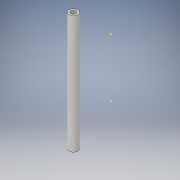
# Autodesk Inventor part: stem1
Saved by Autodesk Inventor 2019 (Build 230136000, 136)
## iProperties
Created: 2020-02-19
Part Number: stem1
Material: Generic
Document SubType Name: Modeling
Designer: FCI-L628
Density: 1 g/cm^3
Appearance: Default
Author: FCI-L628
Autodesk Inventor part; units mm, degrees
ref_plane "YZ Plane" through (0, 0, 0) normal (1, 0, 0) x (0, 1, 0)
ref_plane "XZ Plane" through (0, 0, 0) normal (0, 1, 0) x (-1, 0, 0)
ref_plane "XY Plane" through (0, 0, 0) normal (0, 0, 1) x (1, 0, 0)
sketch "Sketch1" plane through (0, 0, 0) normal (0, 0, 1) x (1, 0, 0)
  point P0 (0, 0)
sketch "Sketch2" plane through (0, 0, 0) normal (0, 0, 1) x (1, 0, 0)
  line L0 (-9.2557, 14.4492) -> (-8.1759, 14.4492)
  line L1 (-8.1759, 14.4492) -> (-8.1759, -14.7063)
  line L2 (-8.1759, -14.7063) -> (-9.2557, -14.7063)
  line L3 (-9.2557, -14.7063) -> (-9.2557, 14.4492)
  point P0 (0, 0)
  constraints: 8 end point, 2 parallel, 1 horizontal, 1 perpendicular
revolve "Revolution1" add sketch "Sketch2" angle 360 about axis through (-9.2557, -14.7063, 0) along (0, 1, 0)
sketch "Sketch3" plane through (-9.2557, 14.4492, 0) normal (0, 1, 0) x (1, 0, 0)
  circle A0 centre (0, 0) radius 1.0798 projected
  circle A1 centre (0, 0) radius 0.6277
  point P0 (9.2557, 0)
  constraints: 1 centre point, 1 coincident
sketch "Sketch4" plane through (-9.2557, 14.4492, 0) normal (0, 1, 0) x (1, 0, 0)
  point P0 (9.2557, 0)
extrude "Extrusion1" cut sketch "Sketch3" against normal blind 25.4 contours A1
body "Solid1"
